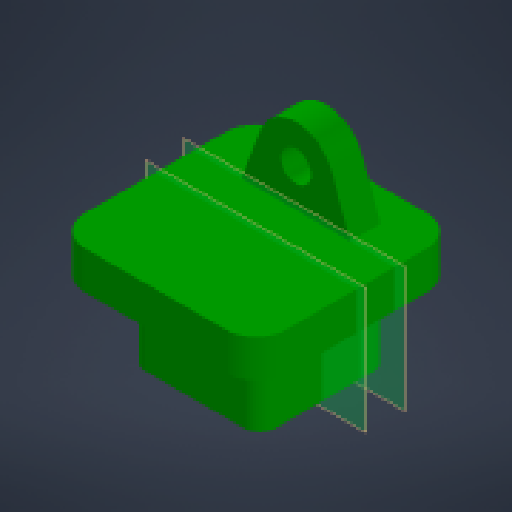
# Autodesk Inventor part: cum_holder_down
Saved by Autodesk Inventor 2024 (Build 280153000, 153)
## iProperties
Created: 2023-05-16
Part Number: cum_holder_down
Material: Типовые
Document SubType Name: Modeling
Designer: user
Density: 1 g/cm^3
Appearance: По умолчанию
Author: user
Autodesk Inventor part; units mm, degrees
ref_plane "YZ Plane" through (0, 0, 0) normal (1, 0, 0) x (0, 1, 0)
ref_plane "XZ Plane" through (0, 0, 0) normal (0, 1, 0) x (-1, 0, 0)
ref_plane "XY Plane" through (0, 0, 0) normal (0, 0, 1) x (1, 0, 0)
sketch "Эскиз1" plane through (0, 0, 0) normal (0, 0, 1) x (1, 0, 0)
  line L0 (8.5, -8.5) -> (-8.5, -8.5) projected
  line L1 (8.5, 8.5) -> (8.5, -8.5) projected
  line L2 (-8.5, -8.5) -> (-8.5, 8.5) projected
  line L3 (-8.5, 8.5) -> (8.5, 8.5) projected
  line L4 (-6.5, -6.5) -> (6.5, -6.5)
  line L5 (6.5, -6.5) -> (6.5, 6.5)
  line L6 (6.5, 6.5) -> (-6.5, 6.5)
  line L7 (-6.5, 6.5) -> (-6.5, -6.5)
  point P0 (0, 0)
  dimension "d0" = 2
  constraints: 8 end point, 3 other
  measures "d0" distance between parallel lines of L0 L4
extrude "Выдавливание1" add sketch "Эскиз1" against normal blind 10
sketch "Эскиз2" plane through (0, 0, 0) normal (0, 0, 1) x (1, 0, 0)
  line L0 (13, -13.5) -> (-13.5, -13.5) projected
  line L1 (13, 13) -> (13, -13.5) projected
  line L2 (-13.5, 13) -> (13, 13) projected
  line L3 (-13.5, -13.5) -> (-13.5, 13) projected
  point P0 (0, 0)
extrude "Выдавливание2" add sketch "Эскиз2" along normal blind 5
fillet "Сопряжение1" radius 2 4 edges at (8.5, 8.5, -5) (-8.5, 8.5, -5) (-8.5, -8.5, -5) (8.5, -8.5, -5)
fillet "Сопряжение2" radius 4 4 edges at (-13.5, -13.5, 2.5) (13, -13.5, 2.5) (13, 13, 2.5) (-13.5, 13, 2.5)
ref_plane "РабПлоскость2" through (-9.5, 4.75, 0) normal (0, 1, 0) x (1, 0, 0)
ref_plane "РабПлоскость1" through (-9.5, -0.25, 0) normal (0, 1, 0) x (1, 0, 0)
sketch "Эскиз3" plane through (-9.5, 4.75, 0) normal (0, 1, 0) x (1, 0, 0)
  line L0 (0, -5) -> (18.5, -5) projected
  line L1 (2.3593, -5) -> (4.8015, -11.7101)
  line L2 (16.6407, -5) -> (14.1985, -11.7101)
  arc A0 (4.8015, -11.7101) -> (14.1985, -11.7101) centre (9.5, -10) ccw
  circle A1 centre (9.5, -10) radius 2
  line L3 (16, 10) -> (3, 10) projected
  line L4 (0, -5) -> (-4, -5) projected
  point P0 (9.5, 0)
  point P1 (9.5, 10)
  dimension "d10" = 4
  dimension "d11" = 5
  dimension "d12" = 5
  dimension "d13" = 70
  constraints: 4 end point, 2 centre point, 2 point on circle, 2 point on line, 2 tangent, 1 coincident, 1 horizontal alignment, 1 midpoint, 1 vertical alignment
  measures "d10" diameter of A1
  measures "d11" radius of A0
  measures "d12" distance from line of A0.centre L4
  measures "d13" angle of L0 L2
extrude "Выдавливание3" add sketch "Эскиз3" along normal blind 4
